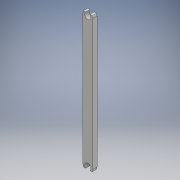
# Autodesk Inventor part: Holder 2
Saved by Autodesk Inventor 2017 (Build 210142000, 142)
## iProperties
Created: 2018-10-03
Part Number: Holder 2
Material: Generic
Document SubType Name: Modeling
Designer: Paulius
Density: 1 g/cm^3
Appearance: Default
Author: Paulius
Autodesk Inventor part; units mm, degrees
ref_plane "YZ Plane" through (0, 0, 0) normal (1, 0, 0) x (0, 1, 0)
ref_plane "XZ Plane" through (0, 0, 0) normal (0, 1, 0) x (-1, 0, 0)
ref_plane "XY Plane" through (0, 0, 0) normal (0, 0, 1) x (1, 0, 0)
sketch "Sketch1" plane through (0, 0, 0) normal (0, 1, 0) x (-1, 0, 0)
  arc A0 (2.4889, -2.6698) -> (-2.4889, -2.6698) centre (0, 0) ccw
  line L0 (2.4889, -2.6698) -> (4.9794, -2.6698)
  line L1 (-4.9794, -2.6698) -> (-2.4889, -2.6698)
  line L2 (-5.65, 0) -> (-5.65, 76)
  line L3 (5.65, 76) -> (5.65, 0)
  arc A1 (-2.4889, 154.6698) -> (2.4889, 154.6698) centre (0, 152) ccw
  line L4 (2.4889, 154.6698) -> (4.9794, 154.6698)
  line L5 (-4.9794, 154.6698) -> (-2.4889, 154.6698)
  line L6 (-5.65, 152) -> (-5.65, 76)
  line L7 (5.65, 76) -> (5.65, 152)
  arc A2 (4.9794, -2.6698) -> (5.65, 0) centre (0, 0) ccw
  arc A3 (-5.65, 0) -> (-4.9794, -2.6698) centre (0, 0) ccw
  arc A4 (-4.9794, 154.6698) -> (-5.65, 152) centre (0, 152) ccw
  arc A5 (5.65, 152) -> (4.9794, 154.6698) centre (0, 152) ccw
  dimension "d5" = 7.3
  dimension "d7" = 76
  constraints: 16 end point, 12 point on circle, 6 centre point, 4 point on line, 2 coincident, 2 tangent, 1 horizontal, 1 vertical
  measures "d5" diameter of A0
  measures "d7" distance of L2.start L2.end
extrude "Extrusion1" add sketch "Sketch1" along normal blind 5
body "Solid1"
